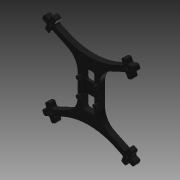
# Autodesk Inventor part: micro_h-quad-naze
Saved by Autodesk Inventor 2014 (Build 180170000, 170)
## iProperties
Created: 2013-01-19
Part Number: micro_h-quad-naze
Material: Plastique ABS
Document SubType Name: Modeling
Designer: Army
Density: 1.06 g/cm^3
Mass: 59.4442 g
Surface Area: 227.74 cm^2
Volume: 56.0794 cm^3
Appearance: Moulé noir
Author: Army
Autodesk Inventor part; units mm, degrees
ref_plane "YZ Plane" through (0, 0, 0) normal (1, 0, 0) x (0, 1, 0)
ref_plane "XZ Plane" through (0, 0, 0) normal (0, 1, 0) x (-1, 0, 0)
ref_plane "XY Plane" through (0, 0, 0) normal (0, 0, 1) x (1, 0, 0)
sketch "Sketch1" plane through (0, 0, 0) normal (0, 1, 0) x (-1, 0, 0)
  line L0 (-10.4875, 33.5925) -> (-10.4875, 0)
  circle A0 centre (-69.85, 69.85) radius 2.5
  circle A1 centre (-15.25, 15.25) radius 1.25
  line L1 (-69.85, 69.85) -> (-28.5605, 50.5964) construction
  line L2 (-85.4573, 71.873) -> (-81.4319, 80.5056)
  line L3 (-18.409, 51.1175) -> (-10.4875, 51.1175)
  circle A2 centre (-76.9328, 73.1528) radius 1
  circle A3 centre (-62.7672, 66.5472) radius 1
  line L4 (-20.0125, 41.3556) -> (-20.0125, 0)
  line L5 (-10.4875, 33.5925) -> (0, 33.5925)
  line L6 (-59.1944, 81.4319) -> (-67.827, 85.4573)
  line L7 (-80.5056, 58.2681) -> (-71.873, 54.2427)
  line L8 (-71.873, 54.2427) -> (-67.5464, 63.521)
  line L9 (-63.521, 72.1536) -> (-59.1944, 81.4319)
  line L10 (-85.4573, 71.873) -> (-76.179, 67.5464)
  line L11 (-67.5464, 63.521) -> (-20.0125, 41.3556)
  line L12 (-81.4319, 80.5056) -> (-72.1536, 76.179)
  line L13 (-63.521, 72.1536) -> (-18.409, 51.1175)
  line L14 (-67.827, 85.4573) -> (-72.1536, 76.179)
  line L15 (-76.179, 67.5464) -> (-80.5056, 58.2681)
  circle A4 centre (-66.5472, 76.9328) radius 1
  circle A5 centre (-73.1528, 62.7672) radius 1
  line L16 (-10.4875, 51.1175) -> (0, 51.1175)
  line L17 (0, 0) -> (0, 51.1175) construction
  line L18 (0, 0) -> (-20.0125, 0) construction
  line L19 (10.4875, 33.5925) -> (10.4875, 0)
  circle A6 centre (69.85, 69.85) radius 2.5
  circle A7 centre (15.25, 15.25) radius 1.25
  line L20 (69.85, 69.85) -> (28.5605, 50.5964) construction
  line L21 (85.4573, 71.873) -> (81.4319, 80.5056)
  line L22 (18.409, 51.1175) -> (10.4875, 51.1175)
  circle A8 centre (76.9328, 73.1528) radius 1
  circle A9 centre (62.7672, 66.5472) radius 1
  line L23 (20.0125, 41.3556) -> (20.0125, 0)
  line L24 (10.4875, 33.5925) -> (0, 33.5925)
  line L25 (59.1944, 81.4319) -> (67.827, 85.4573)
  line L26 (80.5056, 58.2681) -> (71.873, 54.2427)
  line L27 (71.873, 54.2427) -> (67.5464, 63.521)
  line L28 (63.521, 72.1536) -> (59.1944, 81.4319)
  line L29 (85.4573, 71.873) -> (76.179, 67.5464)
  line L30 (67.5464, 63.521) -> (20.0125, 41.3556)
  line L31 (81.4319, 80.5056) -> (72.1536, 76.179)
  line L32 (63.521, 72.1536) -> (18.409, 51.1175)
  line L33 (67.827, 85.4573) -> (72.1536, 76.179)
  line L34 (76.179, 67.5464) -> (80.5056, 58.2681)
  circle A10 centre (66.5472, 76.9328) radius 1
  circle A11 centre (73.1528, 62.7672) radius 1
  line L35 (10.4875, 51.1175) -> (0, 51.1175)
  line L36 (0, 0) -> (20.0125, 0) construction
  line L37 (-10.4875, -33.5925) -> (-10.4875, 0)
  circle A12 centre (-69.85, -69.85) radius 2.5
  circle A13 centre (-15.25, -15.25) radius 1.25
  line L38 (-69.85, -69.85) -> (-28.5605, -50.5964) construction
  line L39 (-85.4573, -71.873) -> (-81.4319, -80.5056)
  line L40 (-18.409, -51.1175) -> (-10.4875, -51.1175)
  circle A14 centre (-76.9328, -73.1528) radius 1
  circle A15 centre (-62.7672, -66.5472) radius 1
  line L41 (-20.0125, -41.3556) -> (-20.0125, 0)
  line L42 (-10.4875, -33.5925) -> (0, -33.5925)
  line L43 (-59.1944, -81.4319) -> (-67.827, -85.4573)
  line L44 (-80.5056, -58.2681) -> (-71.873, -54.2427)
  line L45 (-71.873, -54.2427) -> (-67.5464, -63.521)
  line L46 (-63.521, -72.1536) -> (-59.1944, -81.4319)
  line L47 (-85.4573, -71.873) -> (-76.179, -67.5464)
  line L48 (-67.5464, -63.521) -> (-20.0125, -41.3556)
  line L49 (-81.4319, -80.5056) -> (-72.1536, -76.179)
  line L50 (-63.521, -72.1536) -> (-18.409, -51.1175)
  line L51 (-67.827, -85.4573) -> (-72.1536, -76.179)
  line L52 (-76.179, -67.5464) -> (-80.5056, -58.2681)
  circle A16 centre (-66.5472, -76.9328) radius 1
  circle A17 centre (-73.1528, -62.7672) radius 1
  line L53 (-10.4875, -51.1175) -> (0, -51.1175)
  line L54 (0, 0) -> (0, -51.1175) construction
  line L55 (67.5464, -63.521) -> (20.0125, -41.3556)
  circle A18 centre (62.7672, -66.5472) radius 1
  line L56 (63.521, -72.1536) -> (18.409, -51.1175)
  line L57 (69.85, -69.85) -> (28.5605, -50.5964) construction
  circle A19 centre (66.5472, -76.9328) radius 1
  line L58 (71.873, -54.2427) -> (67.5464, -63.521)
  line L59 (85.4573, -71.873) -> (81.4319, -80.5056)
  line L60 (85.4573, -71.873) -> (76.179, -67.5464)
  line L61 (80.5056, -58.2681) -> (71.873, -54.2427)
  circle A20 centre (73.1528, -62.7672) radius 1
  line L62 (18.409, -51.1175) -> (10.4875, -51.1175)
  line L63 (10.4875, -51.1175) -> (0, -51.1175)
  line L64 (10.4875, -33.5925) -> (0, -33.5925)
  circle A21 centre (15.25, -15.25) radius 1.25
  line L65 (20.0125, -41.3556) -> (20.0125, 0)
  line L66 (10.4875, -33.5925) -> (10.4875, 0)
  circle A22 centre (76.9328, -73.1528) radius 1
  line L67 (76.179, -67.5464) -> (80.5056, -58.2681)
  line L68 (81.4319, -80.5056) -> (72.1536, -76.179)
  line L69 (67.827, -85.4573) -> (72.1536, -76.179)
  line L70 (63.521, -72.1536) -> (59.1944, -81.4319)
  line L71 (59.1944, -81.4319) -> (67.827, -85.4573)
  circle A23 centre (69.85, -69.85) radius 2.5
  line L72 (10.4875, 33.5925) -> (10.4875, -33.5925)
  line L73 (-10.4875, -33.5925) -> (-10.4875, 41.5925)
  point P0 (-69.85, 69.85)
  point P1 (69.85, 69.85)
  point P2 (-69.85, -69.85)
  point P3 (69.85, -69.85)
  dimension "d11" = 5
  dimension "d17" = 2.5
  dimension "d25" = 15.63
  dimension "d27" = 2
  dimension "d28" = 2
  dimension "d56" = 9.525
  dimension "d60" = 9.525
  dimension "d62" = 30
  dimension "d64" = 2
  dimension "d65" = 2
  dimension "d66" = 7.815
  dimension "d67" = 7.815
  dimension "d69" = 33.5925
  dimension "d71" = 17.525
  dimension "d73" = 15.25
  constraints: 148 end point, 71 symmetric about line, 24 centre point, 14 point on line, 6 parallel, 2 perpendicular, 18 other
  measures "d11" diameter of A0
  measures "d17" diameter of A1
  measures "d25" distance of A3.centre A2.centre
  measures "d27" diameter of A3
  measures "d28" diameter of A2
  measures "d56" distance between parallel lines of L0 L4
  measures "d60" distance of L6.end L6.start
  measures "d62" distance between parallel lines of L7 L6
  measures "d64" diameter of A4
  measures "d65" diameter of A5
  measures "d66" distance from line of L1 A4.centre
  measures "d67" distance from line of L1 A5.centre
  measures "d69" distance from line of L5 point (0, 0)
  measures "d71" distance between parallel lines of L3 L5
  measures "d73" vertical distance of L0.end A1.centre
extrude "Extrusion1" add sketch "Sketch1" along normal blind 10
sketch "Sketch2" plane through (0, 10, 0) normal (0, 1, 0) x (1, 0, 0)
  circle A0 centre (15.25, 15.25) radius 1.25 projected
  circle A1 centre (-15.25, 15.25) radius 1.25 projected
  circle A2 centre (-15.25, -15.25) radius 1.25 projected
  circle A3 centre (15.25, -15.25) radius 1.25 projected
  circle A4 centre (-15.25, 15.25) radius 3.5
  circle A5 centre (15.25, 15.25) radius 3.5
  circle A6 centre (15.25, -15.25) radius 3.5
  circle A7 centre (-15.25, -15.25) radius 3.5
  point P0 (0, 0)
  dimension "d31" = 7
  dimension "d34" = 7
  dimension "d35" = 7
  dimension "d36" = 7
  constraints: 4 centre point, 4 coincident
  measures "d31" diameter of A7
  measures "d34" diameter of A6
  measures "d35" diameter of A4
  measures "d36" diameter of A5
extrude "Extrusion2" add sketch "Sketch2" along normal blind 5
sketch "Sketch3" plane through (0, 0, 0) normal (0, -1, 0) x (1, 0, 0)
  circle A0 centre (15.25, -15.25) radius 1.25 projected
  circle A1 centre (-15.25, -15.25) radius 1.25 projected
  circle A2 centre (-15.25, 15.25) radius 1.25 projected
  circle A3 centre (15.25, 15.25) radius 1.25 projected
  point P0 (0, 0)
extrude "Extrusion3" add sketch "Sketch3" against normal blind 4.7625
sketch "Sketch4" plane through (0, 0, 0) normal (0, -1, 0) x (1, 0, 0)
  line L0 (-10.4875, 33.5925) -> (-10.4875, 0)
  circle A0 centre (-69.85, 69.85) radius 2.5
  circle A1 centre (-15.25, 15.25) radius 1.25
  line L1 (-69.85, 69.85) -> (-28.5605, 50.5964) construction
  line L2 (-85.4573, 71.873) -> (-81.4319, 80.5056)
  line L3 (-18.409, 51.1175) -> (-10.4875, 51.1175)
  circle A2 centre (-76.9328, 73.1528) radius 1
  circle A3 centre (-62.7672, 66.5472) radius 1
  line L4 (-20.0125, 41.3556) -> (-20.0125, 0)
  line L5 (-10.4875, 33.5925) -> (0, 33.5925)
  line L6 (-59.1944, 81.4319) -> (-67.827, 85.4573)
  line L7 (-80.5056, 58.2681) -> (-71.873, 54.2427)
  line L8 (-71.873, 54.2427) -> (-67.5464, 63.521)
  line L9 (-63.521, 72.1536) -> (-59.1944, 81.4319)
  line L10 (-85.4573, 71.873) -> (-76.179, 67.5464)
  line L11 (-67.5464, 63.521) -> (-20.0125, 41.3556)
  line L12 (-81.4319, 80.5056) -> (-72.1536, 76.179)
  line L13 (-63.521, 72.1536) -> (-18.409, 51.1175)
  line L14 (-67.827, 85.4573) -> (-72.1536, 76.179)
  line L15 (-76.179, 67.5464) -> (-80.5056, 58.2681)
  circle A4 centre (-66.5472, 76.9328) radius 1
  circle A5 centre (-73.1528, 62.7672) radius 1
  line L16 (-10.4875, 51.1175) -> (0, 51.1175)
  line L17 (0, 0) -> (0, 51.1175) construction
  line L18 (0, 0) -> (-20.0125, 0) construction
  line L19 (67.5464, 63.521) -> (20.0125, 41.3556)
  circle A6 centre (62.7672, 66.5472) radius 1
  line L20 (63.521, 72.1536) -> (18.409, 51.1175)
  line L21 (69.85, 69.85) -> (28.5605, 50.5964) construction
  circle A7 centre (66.5472, 76.9328) radius 1
  line L22 (71.873, 54.2427) -> (67.5464, 63.521)
  line L23 (85.4573, 71.873) -> (81.4319, 80.5056)
  line L24 (85.4573, 71.873) -> (76.179, 67.5464)
  line L25 (80.5056, 58.2681) -> (71.873, 54.2427)
  circle A8 centre (73.1528, 62.7672) radius 1
  line L26 (0, 0) -> (20.0125, 0) construction
  line L27 (18.409, 51.1175) -> (10.4875, 51.1175)
  line L28 (10.4875, 51.1175) -> (0, 51.1175)
  line L29 (10.4875, 33.5925) -> (0, 33.5925)
  circle A9 centre (15.25, 15.25) radius 1.25
  line L30 (20.0125, 41.3556) -> (20.0125, 0)
  line L31 (10.4875, 33.5925) -> (10.4875, 0)
  circle A10 centre (76.9328, 73.1528) radius 1
  line L32 (76.179, 67.5464) -> (80.5056, 58.2681)
  line L33 (81.4319, 80.5056) -> (72.1536, 76.179)
  line L34 (67.827, 85.4573) -> (72.1536, 76.179)
  line L35 (63.521, 72.1536) -> (59.1944, 81.4319)
  line L36 (59.1944, 81.4319) -> (67.827, 85.4573)
  circle A11 centre (69.85, 69.85) radius 2.5
  circle A12 centre (-73.1528, -62.7672) radius 1
  line L37 (-76.179, -67.5464) -> (-80.5056, -58.2681)
  line L38 (-71.873, -54.2427) -> (-67.5464, -63.521)
  line L39 (-80.5056, -58.2681) -> (-71.873, -54.2427)
  circle A13 centre (-69.85, -69.85) radius 2.5
  circle A14 centre (-62.7672, -66.5472) radius 1
  circle A15 centre (-76.9328, -73.1528) radius 1
  line L40 (-85.4573, -71.873) -> (-76.179, -67.5464)
  circle A16 centre (-66.5472, -76.9328) radius 1
  line L41 (-85.4573, -71.873) -> (-81.4319, -80.5056)
  line L42 (-81.4319, -80.5056) -> (-72.1536, -76.179)
  line L43 (-67.827, -85.4573) -> (-72.1536, -76.179)
  line L44 (-59.1944, -81.4319) -> (-67.827, -85.4573)
  line L45 (0, 0) -> (0, -51.1175) construction
  line L46 (10.4875, -51.1175) -> (0, -51.1175)
  line L47 (10.4875, -33.5925) -> (0, -33.5925)
  line L48 (10.4875, -33.5925) -> (10.4875, 0)
  circle A17 centre (15.25, -15.25) radius 1.25
  line L49 (18.409, -51.1175) -> (10.4875, -51.1175)
  line L50 (20.0125, -41.3556) -> (20.0125, 0)
  circle A18 centre (62.7672, -66.5472) radius 1
  circle A19 centre (69.85, -69.85) radius 2.5
  circle A20 centre (73.1528, -62.7672) radius 1
  circle A21 centre (66.5472, -76.9328) radius 1
  line L51 (80.5056, -58.2681) -> (71.873, -54.2427)
  line L52 (76.179, -67.5464) -> (80.5056, -58.2681)
  line L53 (63.521, -72.1536) -> (59.1944, -81.4319)
  line L54 (59.1944, -81.4319) -> (67.827, -85.4573)
  circle A22 centre (76.9328, -73.1528) radius 1
  line L55 (67.827, -85.4573) -> (72.1536, -76.179)
  line L56 (85.4573, -71.873) -> (76.179, -67.5464)
  line L57 (81.4319, -80.5056) -> (72.1536, -76.179)
  line L58 (85.4573, -71.873) -> (81.4319, -80.5056)
  line L59 (69.85, -69.85) -> (28.5605, -50.5964) construction
  line L60 (63.521, -72.1536) -> (18.409, -51.1175)
  line L61 (67.5464, -63.521) -> (20.0125, -41.3556)
  line L62 (71.873, -54.2427) -> (67.5464, -63.521)
  line L63 (-10.4875, -33.5925) -> (-10.4875, 0)
  circle A23 centre (-15.25, -15.25) radius 1.25
  line L64 (-69.85, -69.85) -> (-28.5605, -50.5964) construction
  line L65 (-18.409, -51.1175) -> (-10.4875, -51.1175)
  line L66 (-67.5464, -63.521) -> (-20.0125, -41.3556)
  line L67 (-63.521, -72.1536) -> (-18.409, -51.1175)
  line L68 (-20.0125, -41.3556) -> (-20.0125, 0)
  line L69 (-10.4875, -33.5925) -> (0, -33.5925)
  line L70 (-10.4875, -51.1175) -> (0, -51.1175)
  line L71 (-63.521, -72.1536) -> (-59.1944, -81.4319)
  line L72 (10.4875, 33.5925) -> (10.4875, -33.5925)
  line L73 (-10.4875, -33.5925) -> (-10.4875, 41.5925)
  point P0 (-69.85, 69.85)
  point P1 (69.85, 69.85)
  point P2 (-69.85, -69.85)
  point P3 (69.85, -69.85)
  dimension "d87" = 5
  dimension "d88" = 2.5
  dimension "d89" = 15.63
  dimension "d90" = 2
  dimension "d91" = 2
  dimension "d92" = 9.525
  dimension "d93" = 9.525
  dimension "d94" = 30
  dimension "d95" = 2
  dimension "d96" = 2
  dimension "d97" = 7.815
  dimension "d98" = 7.815
  dimension "d99" = 33.5925
  dimension "d100" = 17.525
  dimension "d101" = 15.25
  constraints: 148 end point, 71 symmetric about line, 24 centre point, 14 point on line, 6 parallel, 2 perpendicular, 18 other
  measures "d87" diameter of A0
  measures "d88" diameter of A1
  measures "d89" distance of A3.centre A2.centre
  measures "d90" diameter of A3
  measures "d91" diameter of A2
  measures "d92" distance between parallel lines of L0 L4
  measures "d93" distance of L6.end L6.start
  measures "d94" distance between parallel lines of L7 L6
  measures "d95" diameter of A4
  measures "d96" diameter of A5
  measures "d97" distance from line of L1 A4.centre
  measures "d98" distance from line of L1 A5.centre
  measures "d99" distance from line of L5 point (0, 0)
  measures "d100" distance between parallel lines of L3 L5
  measures "d101" vertical distance of L0.end A1.centre
extrude "Extrusion4" add sketch "Sketch4" against normal blind 2 contours A0 | A2 | A3 | A4 | A5 | A6 | A7 | A8 | A10 | A11 | A12 | A13 | A14 | A15 | A16 | A18 | A19 | A20 | A21 | A22
sketch "Sketch5" plane through (0, 0, 0) normal (0, -1, 0) x (1, 0, 0)
  line L0 (10.4875, 33.5925) -> (10.4875, -33.5925) projected
  line L1 (-10.4875, -41.5925) -> (-10.4875, 41.5925) projected
  line L2 (-10.4875, -10.4875) -> (10.4875, -10.4875)
  line L3 (10.4875, -10.4875) -> (10.4875, 10.4875)
  line L4 (10.4875, 10.4875) -> (-10.4875, 10.4875)
  line L5 (-10.4875, 10.4875) -> (-10.4875, -10.4875)
  point P0 (10.4875, -41.5925)
  point P1 (0, 0)
  dimension "d43" = 20.975
  dimension "d45" = 10.4875
  dimension "d86" = 20.975
  constraints: 8 end point, 2 parallel, 2 point on line, 1 horizontal, 1 perpendicular
  measures "d43" distance between parallel lines of L2 L4
  measures "d45" distance from line of L4 point (0, 0)
  measures "d86" distance between parallel lines of L3 L5
extrude "Extrusion5" add sketch "Sketch5" against normal blind 4.7625
fillet "Fillet1" radius 114.3 4 edges at (18.409, 5, 51.1175) (-18.409, 5, 51.1175) (18.409, 5, -51.1175) (-18.409, 5, -51.1175)
fillet "Fillet2" radius 3.175 10 edges at (10.4875, 2.3813, 10.4875) (10.4875, 4.7625, 0) (10.4875, 2.3813, -10.4875) (-10.4875, 4.7625, 0) (-10.4875, 2.3813, -10.4875) (-10.4875, 2.3813, 10.4875) (-10.4875, 5, 33.5925) (10.4875, 5, 33.5925) (10.4875, 5, -33.5925) (-10.4875, 5, -33.5925)
fillet "Fillet3" radius 33.02 4 edges at (20.0125, 5, 41.3556) (20.0125, 5, -41.3556) (-20.0125, 5, 41.3556) (-20.0125, 5, -41.3556)
fillet "Fillet5" radius 2.54 40 edges at (81.4319, 5, 80.5056) (85.4573, 5, 71.873) (72.1536, 5, 76.179) (67.827, 5, 85.4573) (59.1944, 5, 81.4319) (80.5056, 5, 58.2681) (76.179, 5, 67.5464) (63.521, 5, 72.1536) (71.873, 5, 54.2427) (67.5464, 5, 63.521) (72.1536, 5, -76.179) (67.827, 5, -85.4573) (59.1944, 5, -81.4319) (81.4319, 5, -80.5056) (85.4573, 5, -71.873) (76.179, 5, -67.5464) (80.5056, 5, -58.2681) (71.873, 5, -54.2427) (67.5464, 5, -63.521) (63.521, 5, -72.1536) (-72.1536, 5, -76.179) (-81.4319, 5, -80.5056) (-67.827, 5, -85.4573) (-59.1944, 5, -81.4319) (-63.521, 5, -72.1536) (-76.179, 5, -67.5464) (-67.5464, 5, -63.521) (-71.873, 5, -54.2427) (-67.5464, 5, 63.521) (-71.873, 5, 54.2427) (-80.5056, 5, 58.2681) (-76.179, 5, 67.5464) (-85.4573, 5, 71.873) (-81.4319, 5, 80.5056) (-72.1536, 5, 76.179) (-67.827, 5, 85.4573) (-59.1944, 5, 81.4319) (-63.521, 5, 72.1536) (-80.5056, 5, -58.2681) (-85.4573, 5, -71.873)
move or copy body "Déplacer des corps1" bodies to move or copy 1 copy no rotation origin (0, 0, 0) rotation axis (1, 0, 0) rotation angle 90
body "Solid1"
